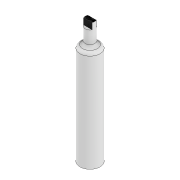
# Autodesk Inventor part: Marker
Saved by Autodesk Inventor 2021 (Build 250183000, 183)
## iProperties
Created: 2022-08-25
Part Number: Marker
Material: PC/ABS Plastic
Document SubType Name: Modeling
Designer: brian
Density: 0.357273 g/cm^3
Appearance: Smooth - White
Mass: 10.1214 g
Surface Area: 67.5683 cm^2
Volume: 28.3297 cm^3
Author: brian
Autodesk Inventor part; units mm, degrees
ref_plane "YZ Plane" through (0, 0, 0) normal (1, 0, 0) x (0, 1, 0)
ref_plane "XZ Plane" through (0, 0, 0) normal (0, 1, 0) x (-1, 0, 0)
ref_plane "XY Plane" through (0, 0, 0) normal (0, 0, 1) x (1, 0, 0)
sketch "Sketch1" plane through (0, 0, 0) normal (0, 1, 0) x (-1, 0, 0)
  circle A0 centre (0, 0) radius 9.5
  dimension "d0" = 19
  constraints: 1 centre point, 1 coincident
  measures "d0" diameter of A0
extrude "Extrusion1" add sketch "Sketch1" along normal blind 96
sketch "Sketch2" plane through (0, 96, 0) normal (0, 1, 0) x (1, 0, 0)
  circle A0 centre (0, 0) radius 4.5
  dimension "d3" = 9
  constraints: 1 centre point, 1 coincident
  measures "d3" diameter of A0
extrude "Extrusion2" add sketch "Sketch2" along normal blind 15
sketch "Sketch3" plane through (0, 111, 0) normal (0, 1, 0) x (1, 0, 0)
  circle A0 centre (0, 0) radius 4.5 projected
  line L0 (-4.5, -2) -> (4.5, -2)
  line L1 (4.5, -2) -> (4.5, 2)
  line L2 (4.5, 2) -> (-4.5, 2)
  line L3 (-4.5, 2) -> (-4.5, -2)
  point P0 (-4.5, 0)
  point P1 (0, 2)
  point P2 (4.0311, 2)
  point P3 (-4.0311, 2)
  point P4 (-4.0311, -2)
  point P5 (4.0311, -2)
  dimension "d6" = 4
  constraints: 8 end point, 2 midpoint, 2 parallel, 1 horizontal, 1 horizontal alignment, 1 perpendicular, 1 tangent, 1 vertical alignment
  measures "d6" distance between parallel lines of L2 L0
extrude "Extrusion3" add sketch "Sketch3" along normal blind 6 contours A0 L0 L2
fillet "Fillet1" radius 3 2 edges at (9.5, 96, 0) (-4.5, 96, 0)
body "Solid1"
